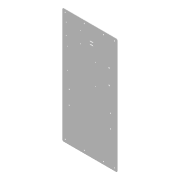
# Autodesk Inventor part: Board_Mounter
Saved by Autodesk Inventor 2020 (Build 240168000, 168)
## iProperties
Created: 2020-11-10
Part Number: Board_Mounter
Material: Generic
Document SubType Name: Modeling
Designer: magnarecta
Density: 1 g/cm^3
Appearance: Default
Author: magnarecta
Autodesk Inventor part; units mm, degrees
ref_plane "YZ Plane" through (0, 0, 0) normal (1, 0, 0) x (0, 1, 0)
ref_plane "XZ Plane" through (0, 0, 0) normal (0, 1, 0) x (-1, 0, 0)
ref_plane "XY Plane" through (0, 0, 0) normal (0, 0, 1) x (1, 0, 0)
sketch "Sketch2" plane through (0, 0, 0) normal (0, 0, 1) x (1, 0, 0)
  line L0 (100, -210) -> (-100, -210)
  line L1 (-100, -210) -> (-100, 210)
  line L2 (-100, 210) -> (100, 210)
  line L3 (100, 210) -> (100, -210)
  line L4 (100, -210) -> (-100, 210) construction
  line L5 (-100, -210) -> (100, 210) construction
  point P0 (0, 0)
  dimension "d4" = 420
  dimension "d5" = 200
  constraints: 12 end point, 2 midpoint, 2 parallel, 1 horizontal, 1 perpendicular
  measures "d4" distance of L2.end L0.start
  measures "d5" distance of L0.start L0.end
extrude "Extrusion2" add sketch "Sketch2" along normal blind 1.5
sketch "Sketch3" plane through (0, 0, 1.5) normal (0, 0, 1) x (1, 0, 0)
  line L0 (-100, 210) -> (-100, -210) projected
  line L1 (-100, -210) -> (100, -210) projected
  line L2 (100, -210) -> (100, 210) projected
  line L3 (100, 210) -> (-100, 210) projected
  line L4 (-90, 200) -> (-90, -200)
  line L5 (-90, -200) -> (90, -200)
  line L6 (90, -200) -> (90, 200)
  line L7 (90, 200) -> (-90, 200)
  point P0 (0, 0)
  point P1 (-20, 200)
  point P2 (-20, -200)
  point P3 (50, 200)
  point P4 (50, -200)
  point P5 (120, 200)
  point P6 (120, -200)
  dimension "d8" = 10
  dimension "d9" = 70
  dimension "d12" = 70
  constraints: 8 end point, 4 coincident, 2 point on line, 1 horizontal, 1 vertical alignment, 7 other
  measures "d8" distance between parallel lines of L3 L7
  measures "d9" distance from line of point (-20, 200) L4
  measures "d12" distance of point (-20, 200) point (50, 200)
hole "Hole1" at (-90, 200, 1.5) at (90, 200, 1.5) at (-90, -200, 1.5) at (90, -200, 1.5) at (-20, 200, 1.5) at (-20, -200, 1.5) at (50, 200, 1.5) at (120, 200, 1.5) at (120, -200, 1.5) at (50, -200, 1.5) direction (0, 0, -1) diameter 4.3 end through all
sketch "Sketch4" plane through (0, 0, 1.5) normal (0, 0, 1) x (1, 0, 0)
  line L0 (-75, -85) -> (75, -85)
  line L1 (75, -85) -> (75, -35)
  line L2 (75, -35) -> (-75, -35)
  line L3 (-75, -35) -> (-75, -85)
  line L4 (-75, -85) -> (75, -35) construction
  line L5 (75, -85) -> (-75, -35) construction
  line L6 (100, -210) -> (100, 210) projected
  line L7 (100, 210) -> (-100, 210) projected
  line L8 (-100, -210) -> (100, -210) projected
  point P0 (0, 0)
  point P1 (0, -60)
  point P2 (0, -60)
  dimension "d24" = 150
  dimension "d25" = 50
  dimension "d35" = 150
  constraints: 12 end point, 3 midpoint, 2 parallel, 1 horizontal, 1 perpendicular, 1 vertical alignment
  measures "d24" distance of L2.end L1.end
  measures "d25" distance of L1.end L0.end
  measures "d35" distance from line of point (0, -60) L8
hole "Hole2" at (-75, -85, 1.5) at (-75, -35, 1.5) at (75, -85, 1.5) at (75, -35, 1.5) direction (0, 0, -1) diameter 4.3 end through all
sketch "Sketch5" plane through (0, 0, 1.5) normal (0, 0, 1) x (1, 0, 0)
  line L0 (-80.925, 21.95) -> (20.925, 21.95)
  line L1 (20.925, 21.95) -> (20.925, 98.05)
  line L2 (20.925, 98.05) -> (-80.925, 98.05)
  line L3 (-80.925, 98.05) -> (-80.925, 21.95)
  line L4 (-80.925, 21.95) -> (20.925, 98.05) construction
  line L5 (20.925, 21.95) -> (-80.925, 98.05) construction
  point P0 (0, 0)
  point P1 (-30, 60)
  dimension "d36" = 101.85
  dimension "d37" = 76.1
  dimension "d38" = 60
  dimension "d97" = 30
  constraints: 12 end point, 2 midpoint, 2 parallel, 1 horizontal, 1 perpendicular
  measures "d36" distance of L2.end L1.end
  measures "d37" distance of L1.end L0.end
  measures "d38" vertical distance of point (-30, 60) point (0, 0)
  measures "d97" horizontal distance of point (-30, 60) point (0, 0)
hole "Hole3" at (-80.925, 98.05, 1.5) at (-80.925, 21.95, 1.5) at (20.925, 21.95, 1.5) at (20.925, 98.05, 1.5) direction (0, 0, -1) diameter 3.2 end through all
sketch "Sketch6" plane through (0, 0, 1.5) normal (0, 0, 1) x (1, 0, 0)
  line L0 (-34, 129) -> (-86, 129)
  line L1 (-86, 129) -> (-86, 171)
  line L2 (-86, 171) -> (-34, 171)
  line L3 (-34, 171) -> (-34, 129)
  line L4 (-34, 129) -> (-86, 171) construction
  line L5 (-86, 129) -> (-34, 171) construction
  point P0 (0, 0)
  point P1 (-60, 150)
  dimension "d48" = 52
  dimension "d49" = 42
  dimension "d50" = 150
  dimension "d51" = 60
  constraints: 12 end point, 2 midpoint, 2 parallel, 1 horizontal, 1 perpendicular
  measures "d48" distance of L1.end L2.end
  measures "d49" distance of L0.end L1.end
  measures "d50" vertical distance of point (-60, 150) point (0, 0)
  measures "d51" horizontal distance of point (-60, 150) point (0, 0)
hole "Hole4" at (-34, 129, 1.5) at (-34, 171, 1.5) at (-86, 129, 1.5) at (-86, 171, 1.5) direction (0, 0, -1) diameter 3.2 end through all
sketch "Sketch7" plane through (0, 0, 1.5) normal (0, 0, 1) x (1, 0, 0)
  circle A0 centre (-86, 129) radius 1.6 projected
  circle A1 centre (-34, 129) radius 1.6 projected
  circle A2 centre (-34, 171) radius 1.6 projected
  circle A3 centre (-86, 171) radius 1.6 projected
  circle A4 centre (20.925, 21.95) radius 1.6 projected
  circle A5 centre (20.925, 98.05) radius 1.6 projected
  circle A6 centre (75, -85) radius 2.15 projected
  circle A7 centre (75, -35) radius 2.15 projected
  circle A8 centre (50, 200) radius 2.15 projected
  circle A9 centre (-20, 200) radius 2.15 projected
  circle A10 centre (-90, -200) radius 2.15 projected
  circle A11 centre (-90, 200) radius 2.15 projected
  circle A12 centre (90, 200) radius 2.15 projected
  circle A13 centre (90, -200) radius 2.15 projected
  circle A14 centre (-20, -200) radius 2.15 projected
  circle A15 centre (50, -200) radius 2.15 projected
  line L0 (-100, 210) -> (-100, -210) projected
  line L1 (-100, -210) -> (100, -210) projected
  line L2 (100, -210) -> (100, 210) projected
  line L3 (100, 210) -> (-100, 210) projected
  circle A16 centre (-80.925, 21.95) radius 1.6 projected
  circle A17 centre (-80.925, 98.05) radius 1.6 projected
  line L4 (-80.925, 21.95) -> (-80.925, 98.05)
  point P0 (0, 0)
  point P1 (70, 50)
  point P2 (-80.925, 60)
  point P3 (70, 105)
  dimension "d98" = 55
  dimension "d99" = 70
  dimension "d100" = 50
  constraints: 2 end point, 1 midpoint, 1 vertical, 1 vertical alignment
  measures "d98" distance of point (70, 105) point (70, 50)
  measures "d99" horizontal distance of point (70, 105) point (0, 0)
  measures "d100" vertical distance of point (70, 50) point (0, 0)
hole "Hole5" at (70, 50, 1.5) at (70, 105, 1.5) direction (0, 0, -1) diameter 5 end through all
sketch "Sketch9" plane through (0, 0, 1.5) normal (0, 0, 1) x (1, 0, 0)
  circle A0 centre (70, 50) radius 2.5 projected
  circle A1 centre (-86, 129) radius 1.6 projected
  circle A2 centre (-34, 129) radius 1.6 projected
  circle A3 centre (-34, 171) radius 1.6 projected
  circle A4 centre (-86, 171) radius 1.6 projected
  circle A5 centre (20.925, 21.95) radius 1.6 projected
  circle A6 centre (20.925, 98.05) radius 1.6 projected
  circle A7 centre (75, -85) radius 2.15 projected
  circle A8 centre (75, -35) radius 2.15 projected
  circle A9 centre (50, 200) radius 2.15 projected
  circle A10 centre (-20, 200) radius 2.15 projected
  circle A11 centre (-90, -200) radius 2.15 projected
  circle A12 centre (-90, 200) radius 2.15 projected
  circle A13 centre (90, 200) radius 2.15 projected
  circle A14 centre (90, -200) radius 2.15 projected
  circle A15 centre (-20, -200) radius 2.15 projected
  circle A16 centre (50, -200) radius 2.15 projected
  line L0 (-100, 210) -> (-100, -210) projected
  line L1 (-100, -210) -> (100, -210) projected
  line L2 (100, -210) -> (100, 210) projected
  line L3 (100, 210) -> (-100, 210) projected
  line L4 (1.125, 145) -> (10.875, 145) construction
  line L5 (1.125, 143.5) -> (10.875, 143.5)
  line L6 (10.875, 146.5) -> (1.125, 146.5)
  arc A17 (1.125, 146.5) -> (1.125, 143.5) centre (1.125, 145) ccw
  arc A18 (10.875, 143.5) -> (10.875, 146.5) centre (10.875, 145) ccw
  line L7 (10.875, 155) -> (1.125, 155) construction
  line L8 (10.875, 156.5) -> (1.125, 156.5)
  line L9 (1.125, 153.5) -> (10.875, 153.5)
  arc A19 (10.875, 153.5) -> (10.875, 156.5) centre (10.875, 155) ccw
  arc A20 (1.125, 156.5) -> (1.125, 153.5) centre (1.125, 155) ccw
  circle A21 centre (-34, 129) radius 1.6 projected
  circle A22 centre (-34, 171) radius 1.6 projected
  line L10 (-34, 129) -> (-34, 171)
  point P0 (0, 0)
  point P1 (6, 145)
  point P2 (6, 155)
  point P3 (-34, 150)
  dimension "d80" = 1.5
  dimension "d81" = 1.5
  dimension "d82" = 10
  dimension "d83" = 5
  dimension "d84" = 40
  constraints: 18 end point, 8 point on circle, 8 tangent, 4 centre point, 3 midpoint, 3 parallel, 2 vertical alignment, 1 horizontal, 1 vertical
  measures "d80" radius of A19
  measures "d81" radius of A18
  measures "d82" distance between parallel lines of L7 L4
  measures "d83" distance from line of L7 point (-34, 150)
  measures "d84" distance from line of point (6, 155) L10
extrude "Extrusion3" cut sketch "Sketch9" against normal blind 3 contours A17 L6 A18 L5 | A19 L9 A20 L8
fillet "Fillet1" radius 5 4 edges at (100, 210, 0.75) (100, -210, 0.75) (-100, -210, 0.75) (-100, 210, 0.75)
body "Solid2"
